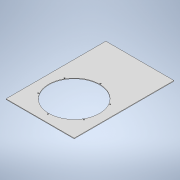
# Autodesk Inventor part: TurnTabletBasePlate
Saved by Autodesk Inventor 2022 (Build 260153000, 153)
## iProperties
Created: 2022-01-15
Part Number: TurnTabletBasePlate
Material: Generic
Document SubType Name: Modeling
Designer: Ty Gazaway
Density: 1 g/cm^3
Appearance: Default
Author: Ty Gazaway
Autodesk Inventor part; units mm, degrees
ref_plane "YZ Plane" through (0, 0, 0) normal (1, 0, 0) x (0, 1, 0)
ref_plane "XZ Plane" through (0, 0, 0) normal (0, 1, 0) x (-1, 0, 0)
ref_plane "XY Plane" through (0, 0, 0) normal (0, 0, 1) x (1, 0, 0)
sketch "Sketch1" plane through (0, 0, 0) normal (0, 1, 0) x (-1, 0, 0)
  line L0 (0, 0) -> (355.6, 0)
  line L1 (355.6, 0) -> (355.6, -520.7)
  line L2 (355.6, -520.7) -> (0, -520.7)
  line L3 (0, -520.7) -> (0, 0)
  circle A0 centre (177.8, -177.8) radius 132.516
  circle A1 centre (177.8, -315.3) radius 3.175
  circle A2 centre (296.8785, -246.55) radius 3.175
  circle A3 centre (296.8785, -109.05) radius 3.175
  circle A4 centre (177.8, -40.3) radius 3.175
  circle A5 centre (58.7215, -109.05) radius 3.175
  circle A6 centre (58.7215, -246.55) radius 3.175
  line L4 (177.8, -177.8) -> (330.2, -177.8) construction
  line L5 (177.8, -177.8) -> (309.7823, -254) construction
  point P0 (177.8, -520.7)
  point P1 (355.6, -260.35)
  dimension "d0" = 355.6
  dimension "d1" = 520.7
  dimension "d2" = 265.032
  dimension "d5" = 177.8
  dimension "d6" = 6.35
  dimension "d7" = 137.5
  dimension "d10" = 360
  dimension "d17" = 152.4
  dimension "d18" = 152.4
  dimension "d19" = 30
  dimension "d22" = 177.8
  constraints: 12 end point, 7 centre point, 2 horizontal, 2 midpoint, 2 parallel, 1 perpendicular, 1 vertical alignment, 13 other
  measures "d0" distance of L1.end L2.end
  measures "d1" distance of L0.end L1.end
  measures "d2" diameter of A0
  measures "d5" distance from line of L1 L4.start
  measures "d6" diameter of A1
  measures "d7" distance of L4.start A1.centre
  measures "d17" distance of L4.start L4.end
  measures "d18" distance of L4.start L5.end
  measures "d19" angle of L4 L5
  measures "d22" distance from line of L0 L4.start
extrude "Extrusion1" add sketch "Sketch1" along normal blind 3.175
body "Solid1"
